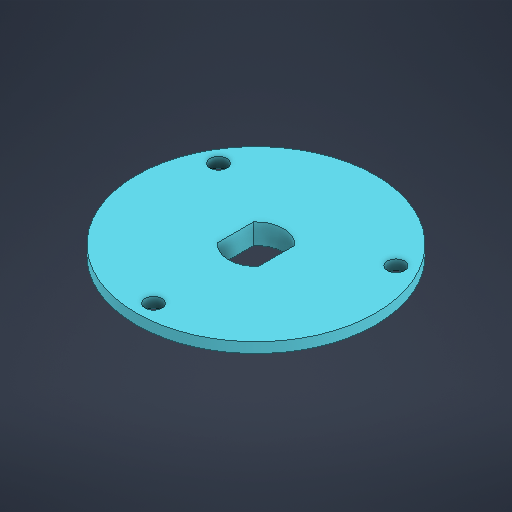
# Autodesk Inventor part: tibea_vodilo_steel
Saved by Autodesk Inventor 2026 (Build 300175000, 175)
## iProperties
Created: 2026-04-25
Part Number: tibea_vodilo_steel
Material: Сталь
Document SubType Name: Modeling
Designer: user
Density: 7.85 g/cm^3
Appearance: Серо-синий
Mass: 122.404 g
Surface Area: 91.3057 cm^2
Volume: 15.5929 cm^3
Author: user
Autodesk Inventor part; units mm, degrees
ref_plane "YZ Plane" through (0, 0, 0) normal (1, 0, 0) x (0, 1, 0)
ref_plane "XZ Plane" through (0, 0, 0) normal (0, 1, 0) x (-1, 0, 0)
ref_plane "XY Plane" through (0, 0, 0) normal (0, 0, 1) x (1, 0, 0)
sketch "Эскиз1" plane through (0, 0, 0) normal (0, 1, 0) x (-1, 0, 0)
  line L0 (48.4444, -57.9334) -> (48.4444, -47.3504) projected
  arc A0 (60.4444, -47.3504) -> (48.4444, -47.3504) centre (54.4444, -52.6419) ccw projected
  line L1 (60.4444, -47.3504) -> (60.4444, -57.9334) projected
  arc A1 (48.4444, -57.9334) -> (60.4444, -57.9334) centre (54.4444, -52.6419) ccw projected
  circle A2 centre (54.4444, -52.6419) radius 30 construction
  circle A3 centre (54.4444, -52.6419) radius 35
  circle A4 centre (28.4636, -67.6419) radius 2.5
  circle A5 centre (54.4444, -52.6419) radius 30 construction
  circle A6 centre (80.4251, -67.6419) radius 2.5
  circle A7 centre (54.4444, -52.6419) radius 30 construction
  circle A8 centre (54.4444, -22.6419) radius 2.5
  point P0 (0, 0)
  point P1 (109.6501, -75.8137)
  dimension "d5" = 60
  dimension "d4" = 70
  dimension "d6" = 5
  dimension "d9" = 360
  constraints: 4 centre point, 2 coincident, 2 vertical alignment, 21 other
  measures "d4" diameter of A3
  measures "d6" diameter of A4
extrude "Выдавливание1" add sketch "Эскиз1" along normal blind 3
sketch "Эскиз4" plane through (-54.4444, 0, -52.6419) normal (0, -1, 0) x (1, 0, 0)
  circle A0 centre (0, 0) radius 35 projected
  circle A1 centre (0, 30) radius 2.5 projected
  circle A2 centre (-25.9808, -15) radius 2.5 projected
  circle A3 centre (25.9808, -15) radius 2.5 projected
  line L0 (-6, 5.2915) -> (-6, -5.2915) projected
  arc A4 (6, 5.2915) -> (-6, 5.2915) centre (0, 0) ccw projected
  line L1 (6, -5.2915) -> (6, 5.2915) projected
  arc A5 (-6, -5.2915) -> (6, -5.2915) centre (0, 0) ccw projected
  circle A6 centre (0, 0) radius 17.5
  point P0 (54.4444, 52.6419)
  dimension "d14" = 35
  constraints: 1 centre point, 1 coincident
  measures "d14" diameter of A6
extrude "Выдавливание3" add sketch "Эскиз4" along normal blind 3 contours A6
equation "\"d2\" = thickness_steel"
equation "\"d15\" = thickness_steel"
equation "\"d17\" = 2 * thickness_steel"
equation "\"tolerance_plazma\" = 0.1"
equation "\"thickness_steel\" = 3"
equation "\"d_main_screw_holes\" = 6.1"
equation "\"d_main_shaft\" = 16"
equation "\"thickness_profile_tibea\" = 4"
equation "\"thickness_profile_femur\" = 3"
equation "\"width_shaft_shift\" = 35"
equation "\"width_flattened_surface\" = 12"
